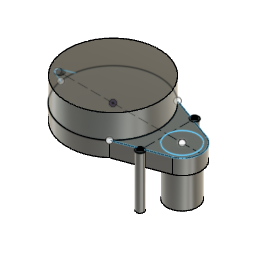
K1D v5 (Autodesk Fusion 360 archive; units mm, degrees)
design "YDLidar X2 approximation"
Autodesk Fusion 360 part; units mm, degrees
note: some values were not read from the file. Chosen so that the rebuilt part matches the saved one: which bodies a step acts on; which face or edge a step refers to.
sketch "Sketch1" plane through (0, 0, 0) normal (0, 0, 1) x (1, 0, 0)
  circle A0 centre (0, 0) radius 30.25
  line L0 (0, 0) -> (-35.3, 0) construction
  line L1 (0, 0) -> (36, 0) construction
  circle A1 centre (-35.3, 0) radius 2.5
  line L2 (36, 0) -> (36, -18) construction
  line L3 (36, 0) -> (36, 18) construction
  circle A2 centre (36, 18) radius 2.5
  circle A3 centre (36, -18) radius 2.5
  line L4 (36, 0) -> (58.2, 0) construction
  line L5 (-29.8847, 4.6871) -> (-37.25, 1.5644)
  line L6 (-29.8847, -4.6871) -> (-37.25, -1.5644)
  arc A4 (-37.25, 1.5644) -> (-37.25, -1.5644) centre (-36.5868, 0) ccw
  arc A5 (50.8692, -11.2997) -> (50.8692, 11.2997) centre (45.8258, 0) ccw
  line L7 (20.1876, 22.5283) -> (33.525, 17.6472)
  line L8 (37.6626, 16.133) -> (50.8692, 11.2997)
  line L9 (20.1876, -22.5283) -> (33.525, -17.6472)
  line L10 (37.6626, -16.133) -> (50.8692, -11.2997)
  circle A6 centre (45.8258, 0) radius 10
  dimension "d1" = 60.5
  dimension "d2" = 35.3
  dimension "d3" = 36
  dimension "d4" = 5
  dimension "d5" = 18
  dimension "d6" = 18
  dimension "d7" = 5
  dimension "d8" = 5
  dimension "d9" = 22.2
  dimension "d10" = 8
  dimension "d13" = 20
  constraint coincident A0.centre L0.start
  constraint horizontal L0
  constraint parallel L0 L1
  constraint coincident L0.end A1.centre
  constraint perpendicular L1 L2
  constraint perpendicular L1 L3
  constraint coincident L3.end A2.centre
  constraint coincident L2.end A3.centre
  constraint perpendicular L3 L4
  constraint coincident A0 L5.start
  constraint symmetric L0 L5.start L6.start
  constraint symmetric L0 L5.end L6.end
  constraint tangent L5 A4
  constraint tangent L6 A4
  constraint coincident A0 L7.start
  constraint symmetric L4 L7.start L9.start
  constraint symmetric L4 A5.end A5.start
  constraint coincident L4.end A5
  constraint coincident A2 L7.end
  constraint collinear L7 L8
  constraint coincident A2 L8.start
  constraint coincident A3 L9.end
  constraint collinear L9 L10
  constraint coincident A3 L10.start
  constraint coincident A1 L5.end
  constraint concentric A5 A6
  measures "d1" diameter of A0
  measures "d2" distance of A0.centre L0.end
  measures "d3" distance of A0.centre L1.end
  measures "d4" diameter of A1
  measures "d5" distance of L1.end L2.end
  measures "d6" distance of L1.end L3.end
  measures "d7" diameter of A2
  measures "d8" diameter of A3
  measures "d9" distance of L1.end L4.end
  measures "d10" distance of L5.start L5.end
  measures "d13" diameter of A6
extrude "Extrude1" add sketch "Sketch1" along normal blind 15.8 contours A0 makes body 1
extrude "Extrude2" add sketch "Sketch1" against normal blind 32 separate body contours A6 makes body 2
extrude "Extrude3" add sketch "Sketch1" against normal blind 30.6 separate body contours A2 | A3 | A1 L5 L6 makes body 3 at (-33.8177, -2.0132, -20.4) makes body 4 at (38.4876, -17.7511, -10.2) makes body 5 at (38.4876, 18.2489, -10.2)
delete_face "DeleteFace1" 1 faces at (-35.7958, 2.181, -10.2) on bodies 3
delete_face "DeleteFace2" 1 faces at (-35.7958, -2.181, -10.2) on bodies 3
move_body "Move1" bodies 3 4 5 to x (1, 0, 0) y (0, 1, 0) z (0, 0, 1) at (0, 0, -3.9)
extrude "Extrude4" add sketch "Sketch1" against normal blind 10 contours A0 A2 A3 A5 L7 L8 L9 L10 | A0 A1 L5 L6 bodies 2 1 3 4 5
extrude "Extrude5" add 3 faces at (-34.7396, 0.6435, -3.9) (37.3366, -18.5849, -3.9) (36.7741, 18.8349, -3.9) along direction (0, 0, 1) blind 3.9 on bodies 2 bodies 2
extrude "Extrude6" add sketch "Sketch1" against normal blind 10 contours A0 bodies 2
extrude "Extrude7" add sketch "Sketch1" against normal blind 10 contours A1 A4 bodies 2
extrude "Extrude8" cut sketch "Sketch1" against normal blind 10 contours A1 L5 | A1 L6 bodies 2

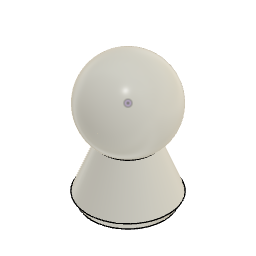
design "Xiaomi 360 camera approximation"
Autodesk Fusion 360 part; units mm, degrees
sketch "Sketch1" plane through (0, 0, 0) normal (0, 0, 1) x (1, 0, 0)
  circle A0 centre (0, 0) radius 37.5
  dimension "d1" = 75
  constraint coincident A0.centre origin
  measures "d1" diameter of A0
ref_plane "WorkPlane1" through (0, 0, 40) normal (0, 0, 1) x (1, 0, 0)
ref_plane "WorkPlane2" through (0, 0, -7) normal (0, 0, 1) x (1, 0, 0)
sketch "Sketch2" plane through (0, 0, -7) normal (0, 0, 1) x (1, 0, 0)
  circle A0 centre (0, 0) radius 33.5
  dimension "d4" = 67
  constraint coincident A0.centre origin
  measures "d4" diameter of A0
ref_plane "WorkPlane3" through (0, 0, 70.5) normal (0, 0, 1) x (1, 0, 0)
sketch "Sketch3" plane through (0, 0, 70.5) normal (0, 0, 1) x (1, 0, 0)
sphere "SpherePrimitive1" add diameter 75 placed x (1, 0, 0) y (0, 1, 0) z (0, 0, 1) at (0, 0, 70.5) makes body 1
sketch "Sketch4" plane through (0, 0, 40) normal (0, 0, 1) x (1, 0, 0)
split "Split1" by plane through (0, 0, 40) normal (0, 0, 1) bodies 1 makes body 2 at (-18.731, -32.4431, 68.8128)
loft "Loft1" add profiles "Sketch1" section 1 section 2 face at (-9.7888, 3.1554, 40) on bodies 2 bodies 2
loft "Loft2" add profiles "Sketch2" section 1 face at (8.8919, -13.3334, 0) section 2 on bodies 2 bodies 2
hidden bodies 1
